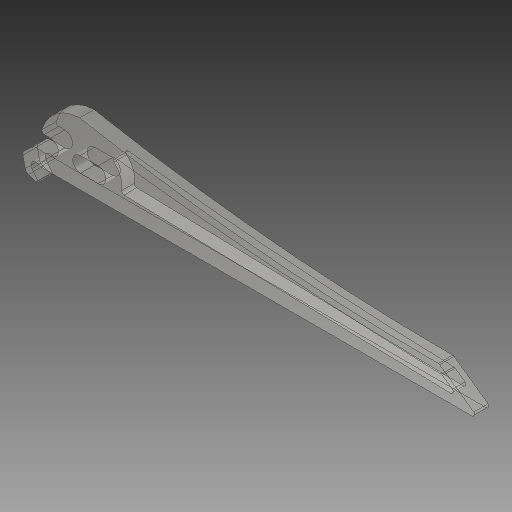
# Autodesk Inventor part: ウイング1
Saved by Autodesk Inventor 2020 (Build 240168000, 168)
## iProperties
Created: 2018-12-14
Part Number: ウイング1
Material: ポリカーボネート、クリア
Document SubType Name: Modeling
Designer: 雪村
Mass: 14.7154 g
Surface Area: 101.427 cm^2
Volume: 12.2628 cm^3
Density: 1.2 g/cm^3
Appearance: ポリカーボネート - クリア
Description: ポリカ 6t
Author: 雪村
Autodesk Inventor part; units mm, degrees
ref_plane "YZ Plane" through (0, 0, 0) normal (1, 0, 0) x (0, 1, 0)
ref_plane "XZ Plane" through (0, 0, 0) normal (0, 1, 0) x (-1, 0, 0)
ref_plane "XY Plane" through (0, 0, 0) normal (0, 0, 1) x (1, 0, 0)
sketch "スケッチ4" plane through (0, 0, 0) normal (0, 0, 1) x (1, 0, 0)
  arc A0 (0, -3.25) -> (0, 3.25) centre (0, 0) ccw
  circle A1 centre (-7.5, 0) radius 3.25 construction
  arc A2 (12.5, 3.25) -> (12.5, -3.25) centre (12.5, 0) ccw
  arc A3 (20, -3.25) -> (20, 3.25) centre (20, 0) ccw
  arc A4 (12.5, 20) -> (-7.5, 0) centre (12.5, 0) ccw construction
  line L0 (12.5, 3.25) -> (20, 3.25)
  line L1 (20, -3.25) -> (12.5, -3.25)
  arc A5 (12.5, 16.75) -> (12.211, 16.7475) centre (12.5, 0) ccw construction
  circle A6 centre (12.5, 20) radius 3.25 construction
  line L2 (0, 3.25) -> (-3.9317, 3.25)
  line L3 (-7.5, -3.25) -> (-4.25, -3.25) construction
  line L4 (20, 9.25) -> (12.5, 9.25)
  arc A7 (12.5, 9.25) -> (12.5, -9.25) centre (12.5, 0) ccw construction
  line L5 (12.5, -9.25) -> (20, -9.25)
  arc A8 (20, -9.25) -> (20, 9.25) centre (20, 0) ccw
  line L6 (-3.9317, 3.25) -> (-7.5, 3.25) construction
  line L7 (-4.25, 0) -> (-4.25, -3.25) construction
  line L8 (-4.25, -3.25) -> (0, -3.25)
  arc A9 (-3.9317, 3.25) -> (-4.25, 0) centre (12.5, 0) ccw construction
  line L9 (-4.25, -3.25) -> (-4.25, -9.25)
  line L10 (-4.25, -9.25) -> (12.5, -9.25)
  line L11 (20, -9.25) -> (180, -9.25)
  line L12 (180, -9.25) -> (162.8622, 2.75)
  line L13 (162.8622, 2.75) -> (162.8622, -9.25) construction
  arc A10 (11.9, 16.8059) -> (12.211, 16.7475) centre (162.8622, 820.4571) ccw construction
  arc A11 (12.211, 16.7475) -> (162.8622, 2.75) centre (162.8622, 820.4571) ccw
  arc A12 (12.211, 16.7475) -> (-3.9317, 3.25) centre (12.5, 0) ccw
  dimension "d39" = 6.5
  dimension "d40" = 6.5
  dimension "d41" = 6.5
  dimension "d42" = 6.5
  dimension "d43" = 7.5
  dimension "d44" = 7.5
  dimension "d46" = 20
  dimension "d47" = 6
  dimension "d48" = 160
  dimension "d49" = 35
  dimension "d50" = 12
  constraints: 28 end point, 27 point on circle, 13 centre point, 13 tangent, 4 horizontal, 3 coincident, 3 horizontal alignment, 3 vertical, 2 line through centre, 1 point on line, 1 vertical alignment, 3 other
  measures "d39" diameter of A0
  measures "d40" diameter of A1
  measures "d41" diameter of A2
  measures "d42" diameter of A3
  measures "d43" distance of point (0, 0) A1.centre
  measures "d44" distance of A3.centre A2.centre
  measures "d46" distance of A3.centre point (0, 0)
  measures "d47" distance between parallel lines of L0 L4
  measures "d48" distance of L5.end L11.end
  measures "d49" angle of L11 L12
  measures "d50" distance of L12.end L13.end
extrude "押し出し3" add sketch "スケッチ4" along normal blind 6
sketch "スケッチ5" plane through (0, 0, 6) normal (0, 0, 1) x (1, 0, 0)
  line L0 (-4.25, -9.25) -> (-5.2687, -8.707)
  line L1 (-7.8081, -11.6738) -> (-5.4042, -14.8709)
  arc A0 (-10.6231, -13.074) -> (-9.2864, -14.5617) centre (-8.6663, -12.6602) ccw
  arc A1 (-5.9588, -15.6467) -> (-5.4042, -14.8709) centre (-5.8038, -15.1714) ccw
  line L2 (-5.9588, -15.6467) -> (-9.2864, -14.5617)
  arc A2 (-10.934, -6.7699) -> (-11.554, -8.6713) centre (-9.5973, -8.2576) ccw
  line L3 (-10.6231, -13.074) -> (-11.554, -8.6713)
  line L4 (-10.934, -6.7699) -> (-7.5867, -3.7623)
  arc A3 (-5.2687, -8.707) -> (-7.8081, -11.6738) centre (-6.2095, -10.4719) ccw
  arc A4 (-6.25, -3.25) -> (-7.5867, -3.7623) centre (-6.25, -5.25) ccw
  line L5 (-6.25, -3.25) -> (-4.25, -3.25)
  line L6 (-4.25, -3.25) -> (-4.25, -9.25)
  line L7 (-4.25, -3.25) -> (-4.25, -9.25) projected
  line L8 (0, -3.25) -> (-4.25, -3.25) projected
  point P0 (0, 0)
  dimension "d54" = 2
  dimension "d55" = 2
  dimension "d56" = 4.5
  dimension "d57" = 2
  dimension "d58" = 4.5
  dimension "d59" = 2
  dimension "d60" = 3.5
  dimension "d61" = 0.5
  dimension "d62" = 4
  dimension "d63" = 2
  dimension "d65" = 25
  dimension "d66" = 35
  dimension "d67" = 120
  dimension "d68" = 120
  dimension "d97" = 1.1544
  dimension "d98" = 61.94
  constraints: 14 end point, 10 point on circle, 10 tangent, 5 centre point, 1 collinear
  measures "d54" distance of L5.end L5.start
  measures "d55" radius of A4
  measures "d56" distance of L4.start L4.end
  measures "d57" radius of A2
  measures "d58" distance of L3.start L3.end
  measures "d59" radius of A0
  measures "d60" distance of L2.start L2.end
  measures "d61" radius of A1
  measures "d62" distance of L1.start L1.end
  measures "d63" radius of A3
  measures "d65" angle of L1 L0
  measures "d66" angle of L2 L1
  measures "d67" angle of L2 L3
  measures "d68" angle of L4 L3
  measures "d97" distance of L0.start L0.end
  measures "d98" angle of L6 L0
extrude "押し出し4" add sketch "スケッチ5" against normal blind 6
fillet "フィレット2" radius 1 2 edges at (162.8622, 2.75, 3) (180, -9.25, 3)
sketch "スケッチ6" plane through (0, 0, 6) normal (0, 0, 1) x (1, 0, 0)
  arc A0 (12.211, 16.7475) -> (162.5472, 2.7501) centre (162.8622, 820.4571) ccw projected
  line L0 (-4.25, -9.25) -> (176.8284, -9.25) projected
  arc A1 (20, -3.25) -> (20, 3.25) centre (20, 0) ccw projected
  line L1 (12.5, 3.25) -> (20, 3.25) projected
  line L2 (20, -3.25) -> (12.5, -3.25) projected
  line L3 (177.402, -7.4308) -> (163.1204, 2.5692) projected
  arc A2 (176.8284, -9.25) -> (177.402, -7.4308) centre (176.8284, -8.25) ccw projected
  arc A3 (163.1204, 2.5692) -> (162.5472, 2.7501) centre (162.5468, 1.7501) ccw projected
  line L4 (163.3443, -1.2499) -> (170.4852, -6.25)
  arc A4 (12.211, 10.7475) -> (26.5915, 8.9414) centre (206.3266, 1498.1342) ccw construction
  line L5 (12.5, -2.25) -> (28.858, -2.6642) construction
  line L6 (163.3443, -1.2499) -> (163.3443, 2.7501)
  line L7 (12.5, 9.25) -> (20, 9.25) construction
  arc A5 (20, -9.25) -> (28.858, -2.6642) centre (20, 0) ccw construction
  line L8 (20, -9.25) -> (12.5, -9.25)
  arc A6 (26.5915, 8.9414) -> (25.8403, 7.1731) centre (26.4717, 7.9486) ccw
  arc A7 (28.858, -2.6642) -> (25.8403, 7.1731) centre (20, 0) ccw
  line L9 (28.858, -2.6642) -> (170.4852, -6.25)
  arc A8 (26.5915, 8.9414) -> (163.3443, -1.2499) centre (206.3266, 1498.1342) ccw
  arc A9 (25.8403, 7.1731) -> (20, 9.25) centre (20, 0) ccw construction
  point P0 (0, 0)
  dimension "d73" = 3
  dimension "d74" = 6
  dimension "d75" = 7
  dimension "d76" = 4
  dimension "d77" = 3
  dimension "d80" = 1500
  dimension "d81" = 6
  dimension "d82" = 2
  constraints: 13 point on circle, 12 end point, 6 centre point, 2 tangent, 2 vertical alignment, 1 collinear, 1 parallel, 1 vertical
  measures "d73" distance between parallel lines of L3 L4
  measures "d74" distance of A0.start A4.start
  measures "d75" distance from line of L0 L5.start
  measures "d76" distance of L4.start L6.end
  measures "d77" distance from line of L0 L4.end
  measures "d80" radius of A4
  measures "d81" radial gap between concentric circles of A1 A5
  measures "d82" diameter of A6
extrude "押し出し5" cut sketch "スケッチ6" against normal blind 6
fillet "フィレット3" radius 1 3 edges at (163.3443, -1.2499, 3) (28.858, -2.6642, 3) (170.4852, -6.25, 3)
sketch "スケッチ8" plane through (0, 0, 6) normal (0, 0, 1) x (1, 0, 0)
  arc A0 (26.5915, 8.9414) -> (163.0449, -1.2412) centre (206.3266, 1498.1342) ccw projected
  arc A1 (163.5897, -1.4217) -> (163.0449, -1.2412) centre (163.0161, -2.2408) ccw projected
  line L0 (163.5897, -1.4217) -> (167.7677, -4.3472) projected
  arc A2 (167.1689, -6.166) -> (167.7677, -4.3472) centre (167.1942, -5.1664) ccw projected
  line L1 (167.1689, -6.166) -> (30.0835, -2.6952) projected
  arc A3 (29.1226, -1.5301) -> (30.0835, -2.6952) centre (30.1088, -1.6955) ccw projected
  arc A4 (29.1226, -1.5301) -> (25.8403, 7.1731) centre (20, 0) ccw projected
  arc A5 (26.5915, 8.9414) -> (25.8403, 7.1731) centre (26.4717, 7.9486) ccw projected
  arc A6 (176.8284, -9.25) -> (177.402, -7.4308) centre (176.8284, -8.25) ccw projected
  line L2 (177.402, -7.4308) -> (163.1204, 2.5692) projected
  arc A7 (163.1204, 2.5692) -> (162.5472, 2.7501) centre (162.5468, 1.7501) ccw projected
  arc A8 (12.211, 16.7475) -> (162.5472, 2.7501) centre (162.8622, 820.4571) ccw projected
  arc A9 (12.211, 16.7475) -> (-3.9317, 3.25) centre (12.5, 0) ccw projected
  line L3 (-3.9317, 3.25) -> (0, 3.25) projected
  arc A10 (0, -3.25) -> (0, 3.25) centre (0, 0) ccw projected
  arc A11 (-6.25, -3.25) -> (-7.5867, -3.7623) centre (-6.25, -5.25) ccw projected
  line L4 (-7.5867, -3.7623) -> (-10.934, -6.7699) projected
  arc A12 (-10.934, -6.7699) -> (-11.554, -8.6713) centre (-9.5973, -8.2576) ccw projected
  line L5 (-11.554, -8.6713) -> (-10.6231, -13.074) projected
  arc A13 (-10.6231, -13.074) -> (-9.2864, -14.5617) centre (-8.6663, -12.6602) ccw projected
  line L6 (-9.2864, -14.5617) -> (-5.9588, -15.6467) projected
  arc A14 (-5.9588, -15.6467) -> (-5.4042, -14.8709) centre (-5.8038, -15.1714) ccw projected
  line L7 (-5.4042, -14.8709) -> (-7.8081, -11.6738) projected
  arc A15 (-5.2687, -8.707) -> (-7.8081, -11.6738) centre (-6.2095, -10.4719) ccw projected
  line L8 (-5.2687, -8.707) -> (-4.25, -9.25) projected
  line L9 (-4.25, -9.25) -> (176.8284, -9.25) projected
  line L10 (12.5, 3.25) -> (20, 3.25) projected
  arc A16 (20, -3.25) -> (20, 3.25) centre (20, 0) ccw projected
  line L11 (20, -3.25) -> (12.5, -3.25) projected
  arc A17 (12.5, 3.25) -> (12.5, -3.25) centre (12.5, 0) ccw projected
  line L12 (0, -3.25) -> (-6.25, -3.25) projected
extrude "押し出し6" add sketch "スケッチ8" against normal blind 0.7 contours A0 A1 L0 A2 L1 A3 A4 A5
fillet "フィレット5" radius 1 1 edges at (-3.9317, 3.25, 3)
equation "\"d44\" = d43"
